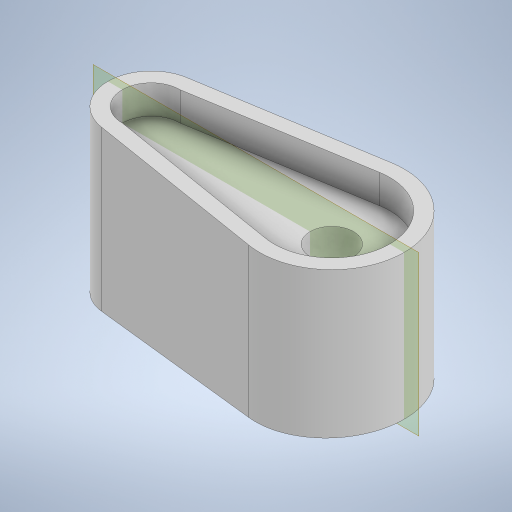
# Autodesk Inventor part: ServoAdapterA
Saved by Autodesk Inventor 2023.1 (Build 271208000, 208)
## iProperties
Created: 2023-04-23
Part Number: ServoAdapterA
Material: Generisch
Document SubType Name: Sheet Metal
Designer: marco
Density: 1 g/cm^3
Sheet Metal Rule: Standard_mm
Appearance: Vorgabe
Author: marco
Autodesk Inventor part; units mm, degrees
ref_plane "YZ Plane" through (0, 0, 0) normal (1, 0, 0) x (0, 1, 0)
ref_plane "XZ Plane" through (0, 0, 0) normal (0, 1, 0) x (-1, 0, 0)
ref_plane "XY Plane" through (0, 0, 0) normal (0, 0, 1) x (1, 0, 0)
sketch "Skizze1" plane through (0, 0, 0) normal (0, 1, 0) x (-1, 0, 0)
  line L0 (0, 0) -> (18.5, 0)
  circle A0 centre (4, 0) radius 4
  circle A1 centre (16.5, 0) radius 2
  line L1 (4.64, 3.9485) -> (16.82, 1.9742)
  line L2 (16.82, -1.9742) -> (4.64, -3.9485)
  circle A2 centre (4, 0) radius 1.5
  circle A3 centre (4, 0) radius 5
  circle A4 centre (16.5, 0) radius 3
  line L3 (4.8, 4.9356) -> (16.98, 2.9614)
  line L4 (16.98, -2.9614) -> (4.8, -4.9356)
  dimension "d0" = 18.5
  dimension "d1" = 8
  dimension "d2" = 4
  dimension "d3" = 3
  dimension "d4" = 10
  dimension "d5" = 6
  constraints: 10 end point, 9 point on circle, 8 tangent, 5 centre point, 3 coincident, 2 point on line, 1 horizontal
  measures "d0" distance of L0.start L0.end
  measures "d1" diameter of A0
  measures "d2" distance of L0.start A0.centre
  measures "d3" diameter of A2
  measures "d4" diameter of A3
  measures "d5" diameter of A4
extrude "Extrusion1" add sketch "Skizze1" along normal blind 1 contours A2 L0 A0 | L0 A0 A2 | A0 L1 A3 L0 | L0 A3 L2 A0 | A3 L1 A4 L0 | L0 A4 L2 A3 | A0 L2 A3 L1 | A4 L1 A1 L0 | L0 A1 L2 A4 | A3 L3 A4 L1 | L2 A4 L4 A3 | A1 L0 | L0 A1 | A4 L2 A1 L1
sketch "Skizze2" plane through (0, 1, 0) normal (0, 1, 0) x (1, 0, 0)
  circle A0 centre (-4, 0) radius 1.5 projected
  circle A1 centre (-4, 0) radius 4
  circle A2 centre (-4, 0) radius 5
  arc A3 (-16.98, 2.9614) -> (-16.98, -2.9614) centre (-16.5, 0) ccw projected
  circle A4 centre (-16.5, 0) radius 3
  circle A5 centre (-16.5, 0) radius 2
  line L0 (-16.5, -2) -> (-4.6485, -3.9471)
  arc A6 (-4.8, -4.9356) -> (-4.8, 4.9356) centre (-4, 0) ccw projected
  line L1 (-16.98, -2.9614) -> (-4.8, -4.9356) projected
  line L2 (-4.8, -4.9356) -> (-16.98, -2.9614)
  line L3 (-16.98, -2.9614) -> (-16.98, 2.9614)
  line L4 (-4.8, 4.9356) -> (-16.98, 2.9614) projected
  line L5 (-4.8, 4.9356) -> (-16.98, 2.9614)
  line L6 (-16.5, 2) -> (-4.6485, 3.9471)
  point P0 (0, 0)
  dimension "d8" = 8
  dimension "d9" = 10
  dimension "d10" = 4
  constraints: 10 end point, 8 point on circle, 4 centre point, 4 coincident, 4 tangent, 1 collinear, 1 point on line
  measures "d8" diameter of A1
  measures "d9" diameter of A2
  measures "d10" diameter of A5
extrude "Extrusion2" add sketch "Skizze2" along normal blind 2 contours A1 L6 A2 L0 | L6 A4 L4 A2 | A2 L1 A4 L0 | L6 A5 L3 A4 | A4 L3 A5 L0 | L3 A5 A3 picked at (-6.3479, 3.8531)
thicken "Verdickung1" operation add thickness 1 both sides no extend neighbours no toward (0, -1, 0) faces at (-13.1533, 0, 0)
sketch "Skizze3" plane through (-4, -1, 0) normal (0, -1, 0) x (1, 0, 0)
  circle A0 centre (0, 0) radius 4
  circle A1 centre (0, 0) radius 5
  arc A2 (-12.98, 2.9614) -> (-12.98, -2.9614) centre (-12.5, 0) ccw projected
  circle A3 centre (-12.5, 0) radius 3
  arc A4 (-0.8, -4.9356) -> (-0.8, 4.9356) centre (0, 0) ccw projected
  line L0 (-0.8, -4.9356) -> (-12.98, -2.9614) projected
  line L1 (-0.8, -4.9356) -> (-12.98, -2.9614)
  line L2 (-12.98, 2.9614) -> (-0.8, 4.9356) projected
  line L3 (-0.8, 4.9356) -> (-12.98, 2.9614)
  point P0 (4, 0)
  dimension "d15" = 8
  constraints: 4 end point, 3 centre point, 3 tangent, 2 coincident, 2 collinear
  measures "d15" diameter of A0
extrude "Extrusion3" add sketch "Skizze3" along normal blind 6
ref_plane "Arbeitsebene1" through (-35.25, -7, 0) normal (0, 0, -1) x (0, -1, 0)
sketch "Skizze4" plane through (-35.25, -7, 0) normal (0, 0, -1) x (0, -1, 0)
  line L0 (0, -18.27) -> (0, -15.75) projected
  line L1 (0, -15.75) -> (0, -36.25)
  line L2 (0, -36.25) -> (-10, -36.25) projected
  line L3 (0, -15.75) -> (0, -36.25)
  line L4 (0, -36.25) -> (0, -30.45) projected
  line L5 (0, -36.25) -> (1.182, -15.75)
  line L6 (0, -36.25) -> (20.534, -36.25) construction
  line L7 (1.182, -15.75) -> (0, -15.75)
  line L8 (0, -15.75) -> (-10, -15.75) projected
  point P0 (-7, -35.25)
  dimension "d18" = 86.7
  constraints: 10 end point, 2 vertical, 1 collinear, 1 equal length, 1 horizontal, 1 point on line
  measures "d18" angle of L6 L5
extrude "Extrusion4" add sketch "Skizze4" along normal mid plane 12
sketch "Skizze5" plane through (-19.5, -7, -6) normal (0, 1, 0) x (1, 0, 0)
  arc A0 (2.52, -3.0386) -> (0, -6) centre (3, -6) ccw projected
  circle A1 centre (3, -6) radius 3
  circle A2 centre (15.5, -6) radius 1.5 projected
  circle A3 centre (15.5, -6) radius 4
  circle A4 centre (15.5, -6) radius 5
  arc A5 (20.5, -6) -> (14.7, -1.0644) centre (15.5, -6) ccw projected
  line L0 (2.52, -3.0386) -> (14.7, -1.0644) projected
  line L1 (14.7, -1.0644) -> (2.52, -3.0386)
  line L2 (14.7, -10.9356) -> (2.52, -8.9614) projected
  line L3 (2.52, -3.0386) -> (2.52, -8.9614)
  line L4 (2.52, -8.9614) -> (14.7, -10.9356)
  line L5 (0, 0) -> (20.5, 0) projected
  line L6 (20.5, -12) -> (0, -12) projected
  line L7 (0, 0) -> (20.5, 0)
  line L8 (20.5, 0) -> (20.5, -12)
  line L9 (20.5, -12) -> (0, -12)
  line L10 (0, -12) -> (0, 0)
  point P0 (19.5, -6)
  point P1 (20.5, -6)
  constraints: 14 end point, 4 equal length, 3 centre point, 3 coincident, 2 point on circle, 2 tangent, 1 horizontal, 1 perpendicular, 1 vertical
extrude "Extrusion5" cut sketch "Skizze5" against normal blind 12 contours A0 L10 L5 L8 A4 L0 | A1 L2 A4 L8 L6 L10 | A2 | A3
equation "\"Biegeradius\" = Stärke"
equation "\"BreiteBiegungsfreistellung\" = Stärke"
equation "\"TiefeBiegungsfreistellung\" = 0.5 * Stärke"
equation "\"GrößeEckenfreistellung\" = 4 * Stärke"
equation "\"MinimalRest\" = 2 * Stärke"
equation "\"Übergangsradius\" = Biegeradius"
equation "\"JacobiRadiusGröße\" = Biegeradius"
equation "\"Abstandsgröße\" = Stärke"
equation "\"Stärke\" = 0.5"
